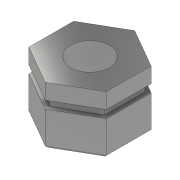
# Autodesk Inventor part: 螺套
Saved by Autodesk Inventor 2022 (Build 260153000, 153)
## iProperties
Created: 2023-03-14
Part Number: 螺套
Material: 不锈钢
Document SubType Name: Modeling
Designer: Lzy18
Density: 8 g/cm^3
Appearance: 半抛光
Author: Lzy18
Autodesk Inventor part; units mm, degrees
ref_plane "YZ Plane" through (0, 0, 0) normal (1, 0, 0) x (0, 1, 0)
ref_plane "XZ Plane" through (0, 0, 0) normal (0, 1, 0) x (-1, 0, 0)
ref_plane "XY Plane" through (0, 0, 0) normal (0, 0, 1) x (1, 0, 0)
sketch "草图1" plane through (0, 0, 0) normal (0, 1, 0) x (-1, 0, 0)
  line L0 (20, -11.547) -> (0, -23.094)
  line L1 (0, -23.094) -> (-20, -11.547)
  line L2 (-20, -11.547) -> (-20, 11.547)
  line L3 (-20, 11.547) -> (0, 23.094)
  line L4 (0, 23.094) -> (20, 11.547)
  line L5 (20, 11.547) -> (20, -11.547)
  point P0 (0, 0)
  point P1 (0, 0)
  dimension "d0" = 40
  constraints: 12 end point, 1 coincident, 13 other
  measures "d0" distance between parallel lines of L2 L5
extrude "拉伸1" add sketch "草图1" along normal mid plane 30
sketch "草图2" plane through (0, 0, 0) normal (0, 0, 1) x (1, 0, 0)
  line L0 (-20, -15) -> (-20, 15) projected
  line L1 (-20, 7) -> (-18, 7)
  line L2 (-18, 7) -> (-18, 3)
  line L3 (-18, 3) -> (-20, 3)
  line L4 (-20, -15) -> (0, -15) projected
  point P0 (0, 0)
  dimension "d3" = 4
  dimension "d4" = 2
  dimension "d5" = 18
  constraints: 6 end point, 2 perpendicular, 2 point on line, 1 horizontal
  measures "d3" distance of L1.end L2.end
  measures "d4" distance between parallel lines of L0 L2
  measures "d5" distance between parallel lines of L4 L3
extrude "拉伸2" cut sketch "草图2" along normal through all both and the other way through all
pattern_circular "环形阵列1" count 6 over 360 about axis through (0, -10, 0) along (0, 1, 0) of "拉伸2"
sketch "草图3" plane through (0, 0, 0) normal (0, 0, 1) x (1, 0, 0)
  line L0 (10, 15) -> (10, -11.5359)
  line L1 (10, -11.5359) -> (16, -15)
  line L2 (20, -15) -> (0, -15) projected
  line L3 (0, 15) -> (20, 15) projected
  line L4 (0, 15) -> (10, 15)
  line L5 (0, 7) -> (0, 15) projected
  line L6 (0, -15) -> (0, 3) projected
  line L7 (0, 15) -> (0, -15)
  line L8 (0, -15) -> (15.0362, -15.0811)
  line L9 (0, -21.0973) -> (0, 21.0162) projected
  point P0 (0, 0)
  dimension "d11" = 60
  dimension "d12" = 10
  dimension "d13" = 16
  constraints: 10 end point, 2 collinear, 1 point on line, 1 vertical
  measures "d11" angle of L6 L1
  measures "d12" distance from line of L0 L3.start
  measures "d13" distance of L1.end L2.end
revolve "旋转1" cut sketch "草图3" angle 360 about axis through (0, -10, 0) along (0, 1, 0)
chamfer "倒角1" distance 1.5 angle 45 6 edges at (10, -15, -17.3205) (20, -15, 0) (10, -15, 17.3205) (-10, -15, 17.3205) (-10, -15, -17.3205) (-20, -15, 0)
